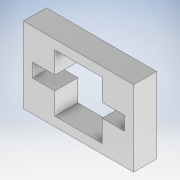
# Autodesk Inventor part: Slot Detector Holder
Saved by Autodesk Inventor 2018 (Build 220112000, 112)
## iProperties
Created: 2018-01-29
Part Number: Slot Detector Holder
Material: ABS Plastic
Document SubType Name: Modeling
Designer: Moochster
Density: 1.06 g/cm^3
Appearance: Smooth - White
Mass: 1.25901 g
Surface Area: 12.0479 cm^2
Volume: 1.18775 cm^3
Author: Moochster
Autodesk Inventor part; units mm, degrees
ref_plane "YZ Plane" through (0, 0, 0) normal (1, 0, 0) x (0, 1, 0)
ref_plane "XZ Plane" through (0, 0, 0) normal (0, 1, 0) x (-1, 0, 0)
ref_plane "XY Plane" through (0, 0, 0) normal (0, 0, 1) x (1, 0, 0)
sketch "Sketch1" plane through (0, 0, 0) normal (0, 1, 0) x (-1, 0, 0)
  line L0 (0, 0) -> (-10.3, 0)
  line L1 (-10.3, 0) -> (-10.3, -12.5)
  line L2 (-10.3, -12.5) -> (0, -12.5)
  line L3 (0, -12.5) -> (0, 0)
  line L4 (6.85, -14.5) -> (-17.15, -14.5)
  line L5 (-17.15, -14.5) -> (-17.15, 2)
  line L6 (-17.15, 2) -> (6.85, 2)
  line L7 (6.85, 2) -> (6.85, -14.5)
  line L8 (0, -7.75) -> (4.85, -7.75)
  line L9 (4.85, -7.75) -> (4.85, -4.75)
  line L10 (4.85, -4.75) -> (0, -4.75)
  line L11 (-10.3, -7.75) -> (-15.15, -7.75)
  line L12 (-15.15, -7.75) -> (-15.15, -4.75)
  line L13 (-15.15, -4.75) -> (-10.3, -4.75)
  point P0 (-15.15, -6.25)
  point P1 (-10.3, -6.25)
  dimension "d0" = 3
  dimension "d1" = 10.3
  dimension "d2" = 12.5
  dimension "d3" = 2
  dimension "d4" = 2
  dimension "d5" = 2
  dimension "d6" = 2
  dimension "d7" = 20
  constraints: 28 end point, 8 point on line, 5 perpendicular, 4 parallel, 3 horizontal, 3 horizontal alignment, 2 midpoint, 1 collinear
  measures "d0" distance of L11.end L12.end
  measures "d1" distance of L0.start L0.end
  measures "d2" distance of L0.end L1.end
  measures "d3" distance between parallel lines of L4 L2
  measures "d4" distance between parallel lines of L0 L6
  measures "d5" distance between parallel lines of L12 L5
  measures "d6" distance between parallel lines of L9 L7
  measures "d7" distance between parallel lines of L9 L12
extrude "Extrusion1" add sketch "Sketch1" along normal blind 5
chamfer "Chamfer1" distance 1 angle 45 2 edges at (-4.85, 5, -6.25) (15.15, 5, -6.25)
body "Solid1"
